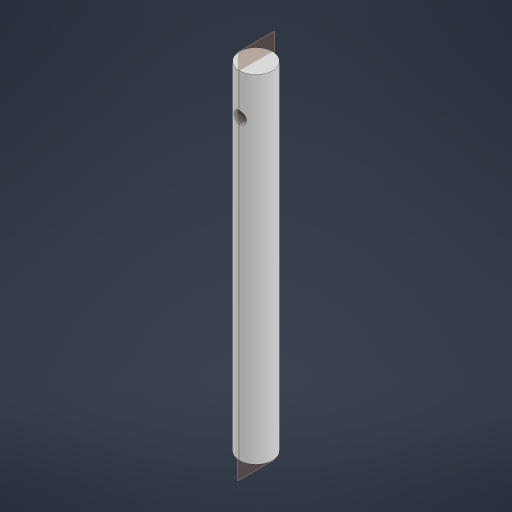
# Autodesk Inventor part: sf_Crankshaft_1
Saved by Autodesk Inventor 2024 (Build 280153000, 153)
## iProperties
Created: 2024-03-20
Part Number: sf_Crankshaft_1
Material: Generisch
Document SubType Name: Modeling
Designer: Simon
Density: 1 g/cm^3
Appearance: Vorgabe
Author: Simon
Autodesk Inventor part; units mm, degrees
ref_plane "XZ Plane" through (0, 0, 0) normal (0, 1, 0) x (-1, 0, 0)
ref_plane "XY Plane" through (0, 0, 0) normal (0, 0, 1) x (1, 0, 0)
sketch "Skizze1" plane through (0, 0, 0) normal (0, 0, 1) x (1, 0, 0)
  circle A0 centre (0, 0) radius 5.5
  dimension "d0" = 11
  constraints: 1 centre point, 1 coincident
  measures "d0" diameter of A0
extrude "Extrusion1" add sketch "Skizze1" along normal mid plane 112.5
sketch "Skizze2" plane through (0, 0, 0) normal (1, 0, 0) x (0, 1, 0)
  line L0 (5.5, -56.25) -> (5.5, 56.25) projected
  line L1 (-5.5, 40.75) -> (5.5, 40.75)
  line L2 (5.5, 40.75) -> (5.5, 44.75)
  line L3 (5.5, 44.75) -> (-5.5, 44.75)
  line L4 (-5.5, 44.75) -> (-5.5, 40.75)
  line L5 (-5.5, 40.75) -> (5.5, 44.75) construction
  line L6 (5.5, 40.75) -> (-5.5, 44.75) construction
  line L7 (-5.5, 44.75) -> (5.5, 44.75)
  line L8 (5.5, 44.75) -> (5.5, 42.75)
  line L9 (5.5, 42.75) -> (-5.5, 42.75)
  line L10 (-5.5, 42.75) -> (-5.5, 44.75)
  point P0 (0, 0)
  point P1 (0, 42.75)
  dimension "d3" = 4
  constraints: 20 end point, 4 parallel, 3 midpoint, 2 horizontal, 2 perpendicular, 1 point on line
  measures "d3" distance of L2.end L1.end
revolve "Umdrehung1" cut sketch "Skizze2" angle 360 about axis through (0, 5.5, 42.75) along (0, -1, 0) contours L9 L4 L3 L0
